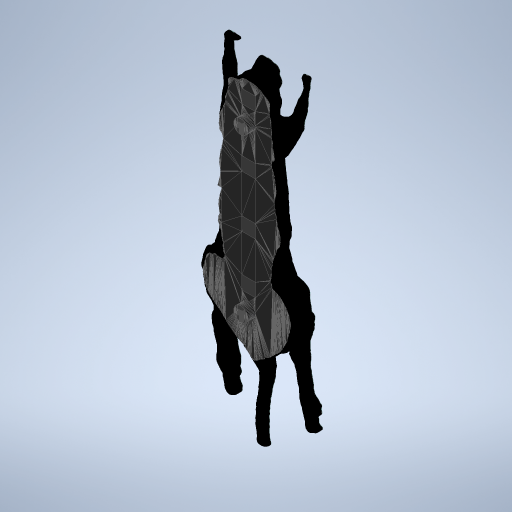
# Autodesk Inventor part: prone_mouse_bottom
Saved by Autodesk Inventor 2023 (Build 270158000, 158)
## iProperties
Created: 2022-12-03
Part Number: prone_mouse_bottom
Material: Generic
Document SubType Name: Modeling
Designer: Admin
Density: 1 g/cm^3
Appearance: Default
Author: Admin
Autodesk Inventor part; units mm, degrees
ref_plane "YZ Plane" through (0, 0, 0) normal (1, 0, 0) x (0, 1, 0)
ref_plane "XZ Plane" through (0, 0, 0) normal (0, 1, 0) x (-1, 0, 0)
ref_plane "XY Plane" through (0, 0, 0) normal (0, 0, 1) x (1, 0, 0)
sketch "Sketch1" plane through (101.5928, 164.0468, 4.5603) normal (0, 0, 1) x (1, 0, 0)
  line L0 (0, 0) -> (-4, 0) projected
  line L1 (0, 0) -> (0, 4) projected
  line L2 (-4, 4) -> (0, 4) projected
  line L3 (-4, 4) -> (-4, 0) projected
  line L4 (0, -17.4194) -> (-4, -17.4194) projected
  line L5 (0, -17.4194) -> (0, -13.4194) projected
  line L6 (0, -13.4194) -> (-4, -13.4194) projected
  line L7 (-4, -13.4194) -> (-4, -17.4194) projected
  line L8 (-4, -32.9752) -> (0, -32.9752) projected
  line L9 (0, -32.9752) -> (0, -28.9752) projected
  line L10 (0, -28.9752) -> (-4, -28.9752) projected
  line L11 (-4, -48.149) -> (-4, -4.9154) projected
  line L12 (0, -44.149) -> (-4, -44.149) projected
  line L13 (0, -48.149) -> (-4, -48.149) projected
  line L14 (0, -13.4194) -> (0, -48.149) projected
  point P0 (-101.5928, -164.0468)
extrude "Extrusion1" add sketch "Sketch1" along normal blind 1.2 contours L0 L3 L2 L1 | L4 L7 L6 L5 | L9 L8 L11 L10 | L14 L13 L11 L12
body "Solid1"
